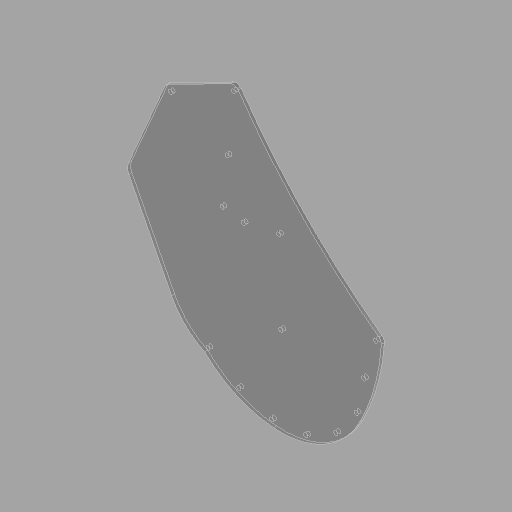
# Autodesk Inventor part: PolyIntakeSides
Saved by Autodesk Inventor 2026.1 (Build 301233000, 233)
## iProperties
Created: 2025-09-20
Part Number: PolyIntakeSides
Material: Polycarbonate, Smoke
Document SubType Name: Modeling
Designer: Teddy
Density: 1.2 g/cm^3
Appearance: Polycarbonate - Smoked
Author: Teddy
Autodesk Inventor part; units mm, degrees
ref_plane "YZ Plane" through (0, 0, 0) normal (1, 0, 0) x (0, 1, 0)
ref_plane "XZ Plane" through (0, 0, 0) normal (0, 1, 0) x (-1, 0, 0)
ref_plane "Work Plane1" through (41.8181, 29.2938, 0) normal (0, 0, 1) x (0.9979, -0.0645, 0)
sketch "Sketch1" plane through (41.8181, 29.2938, 0) normal (0, 0, 1) x (0.9979, -0.0645, 0)
  circle A0 centre (-2.5655, 153.0633) radius 2.0828 projected
  circle A1 centre (-5.319, 89.623) radius 2.1844 projected
  circle A2 centre (-7.5218, 38.8708) radius 2.1844 projected
  circle A3 centre (52.8057, 47.5823) radius 2.1844 projected
  circle A4 centre (-13.5796, -100.6978) radius 2.1844 projected
  circle A5 centre (159.8214, 7.4311) radius 2.1844 projected
  circle A6 centre (-68.0529, 114.1038) radius 2.1844 projected
  arc A7 (-71.2995, 119.5611) -> (-74.0366, 116.2293) centre (-68.0529, 114.1038) ccw
  arc A8 (2.4163, 157.0009) -> (-5.8121, 158.5206) centre (-2.5655, 153.0633) ccw
  arc A9 (161.5237, 1.3135) -> (166.1714, 7.4036) centre (159.8214, 7.4311) ccw construction
  circle A10 centre (52.8057, 47.5823) radius 6.35 construction
  circle A11 centre (-5.319, 89.623) radius 6.35 construction
  circle A12 centre (-7.5218, 38.8708) radius 6.35 construction
  arc A13 (-15.8353, -106.6336) -> (-17.7424, -105.4929) centre (-13.5796, -100.6978) ccw
  line L0 (-71.2995, 119.5611) -> (-5.8121, 158.5206)
  arc A14 (2.4163, 157.0009) -> (163.1954, 12.8105) centre (500.593, 550.7583) ccw
  circle A15 centre (60.913, -39.7814) radius 2.286
  line L1 (-89.9787, 77.2357) -> (7.9234, -87.3286) construction
  line L2 (-83.2674, -13.1743) -> (-114.6948, 39.6521) construction
  arc A16 (161.5237, 1.3135) -> (142.8052, -4.455) centre (256.8502, -341.2711) ccw construction
  arc A17 (-4.6262, -100.2702) -> (-8.8352, -104.9184) centre (256.8502, -341.2711) ccw construction
  arc A18 (4.3909, -99.9458) -> (-4.6262, -100.2702) centre (0.043, -104.5738) ccw construction
  arc A19 (142.8052, -4.455) -> (138.8468, -12.5633) centre (144.8417, -10.4696) ccw construction
  line L3 (-5.7234, -191.6454) -> (22.9273, -174.6006) construction
  arc A20 (4.3909, -99.9458) -> (23.7114, -113.4736) centre (60.913, -39.7814) ccw construction
  line L4 (256.8502, -341.2711) -> (60.913, -39.7814) construction
  line L5 (22.9273, -174.6006) -> (113.5094, -120.7118) construction
  arc A21 (20.8497, -119.1423) -> (149.705, -35.3997) centre (60.913, -39.7814) ccw construction
  arc A22 (17.9881, -124.8109) -> (59.2697, -135.0173) centre (60.913, -39.7814) ccw construction
  arc A23 (24.2841, -113.8012) -> (17.9881, -124.8109) centre (20.8497, -119.1423) ccw construction
  arc A24 (156.0473, -35.0867) -> (143.6088, -37.1771) centre (149.705, -35.3997) ccw construction
  arc A25 (23.7114, -113.4736) -> (143.3627, -35.7126) centre (60.913, -39.7814) ccw construction
  arc A26 (143.3627, -35.7126) -> (138.8468, -12.5633) centre (60.913, -39.7814) ccw construction
  arc A27 (148.2601, -77.7689) -> (166.1714, 7.4036) centre (-49.7266, 8.336) ccw
  arc A28 (148.2601, -77.7689) -> (156.0473, -35.0867) centre (60.913, -39.7814) ccw construction
  arc A29 (166.1714, 7.4036) -> (163.1954, 12.8105) centre (159.8214, 7.4311) ccw
  arc A30 (-17.7424, -105.4929) -> (59.2697, -135.0173) centre (61.3513, -14.3852) ccw
  arc A31 (59.2697, -135.0173) -> (148.2601, -77.7689) centre (60.913, -39.7814) ccw
  arc A32 (-17.7424, -105.4929) -> (-8.8352, -104.9184) centre (-13.5796, -100.6978) ccw construction
  circle A33 centre (20.8497, -119.1423) radius 2.286
  circle A34 centre (56.5923, -128.5764) radius 2.286
  circle A35 centre (93.082, -122.657) radius 2.286
  circle A36 centre (124.0094, -102.4078) radius 2.286
  circle A37 centre (144.0269, -71.3298) radius 2.286
  circle A38 centre (149.6732, -34.7969) radius 2.286
  line L6 (-74.0366, 116.2293) -> (-107.0351, 23.3316)
  line L7 (-105.9822, 12.5873) -> (-54.254, -74.3631)
  arc A39 (-54.254, -74.3631) -> (-15.8353, -106.6336) centre (11.2334, -35.4035) ccw
  line L8 (-89.9787, 77.2357) -> (-91.0414, 74.2438) projected
  arc A40 (-107.0351, 23.3316) -> (-105.9822, 12.5873) centre (-95.0676, 19.0806) ccw
  circle A41 centre (15.4603, 36.6205) radius 2.286
  point P0 (-39.8403, -31.9316)
  point P1 (105.8968, -108.9982)
  point P2 (-109.0311, 17.7123)
  point P3 (-16.8948, -106.2219)
  dimension "d0" = 12.7
  dimension "d3" = 635
  dimension "d6" = 4.572
  dimension "d10" = 355.6
  dimension "d11" = 355.6
  dimension "d12" = 6.35
  dimension "d13" = 69.85
  dimension "d14" = 165.1
  dimension "d15" = 13.97
  dimension "d17" = 6.35
  dimension "d18" = 25.4
  dimension "d19" = 25.4
  dimension "d21" = 215.9
  dimension "d22" = 120.65
  dimension "d23" = 4.572
  dimension "d26" = 120
  dimension "d28" = 6.35
  dimension "d29" = 76.2
  dimension "d30" = 12.7
  dimension "d31" = 4.572
  dimension "d32" = 69.85
  dimension "d33" = 88.9
  constraints: 54 point on circle, 35 centre point, 22 tangent, 12 end point, 10 coincident, 7 equal radius, 4 point on line, 3 parallel, 1 collinear, 12 other
  measures "d0" diameter of A7
  measures "d3" radius of A14
  measures "d6" diameter of A15
  measures "d10" radius of A16
  measures "d11" radius of A17
  measures "d12" radius of A18
  measures "d13" distance from line of L1 A15.centre
  measures "d14" diameter of A20
  measures "d15" distance of point (105.897, -108.998) L5.end
  measures "d17" radius of A23
  measures "d18" distance of A18.centre A21.start
  measures "d19" distance of A19.centre A21.end
  measures "d21" radius of A27
  measures "d22" radius of A30
  measures "d23" diameter of A33
  measures "d28" distance from line of L2 point (-109.031, 17.712)
  measures "d29" radius of A39
  measures "d30" radius of A40
  measures "d31" diameter of A41
  measures "d32" distance from line of A41.centre L1
  measures "d33" distance of A15.centre A41.centre
extrude "Extrusion1" add sketch "Sketch1" along normal blind 3.175 contours A30 A13 A39 | L0 A8 A14 A29 A27 A31 A30 A39 L7 A40 L6 A7
body "Solid1"
